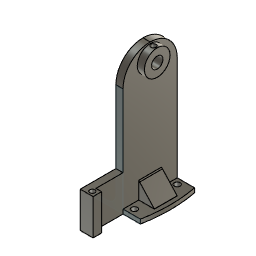
Left handle (Autodesk Fusion 360 design; units mm, degrees)
Autodesk Fusion 360 part; units mm, degrees
note: some values were not read from the file. Set by a fixed rule: which face or edge a step refers to.
sketch "Szkic1" plane through (0, 0, 0) normal (0, 0, 1) x (1, 0, 0)
  circle A0 centre (0, 0) radius 100
  line L0 (66, 19) -> (66, -19)
  line L1 (66, -19) -> (98.1784, -19)
  line L2 (66, 19) -> (98.1784, 19)
  dimension "d1" = 200
  constraint coincident A0.centre origin
  constraint coincident A0 L1.end
  constraint perpendicular L0 L1
  constraint coincident A0 L2.end
  constraint perpendicular L0 L2
  measures "d1" diameter of A0
extrude "Wyciągnięcie proste1" add sketch "Szkic1" along normal blind 3 contours A0 L0 L1 L2 picked at (77.3333, 0)
move_face "Przesuń powierzchnię1" by (-33, 0, 0) 1 faces at (77.3333, 0, 3)
move_body "Przesuń1" bodies 1 to x (1, 0, 0) y (0, 1, 0) z (0, 0, 1) at (-66, 0, 0)
sketch "Szkic2" plane through (0, 0, 3) normal (0, 0, 1) x (-1, 0, 0)
  line L0 (0, 19) -> (-32.1784, 19)
  arc A0 (-32.1784, 19) -> (-32.1784, -19) centre (66, 0) ccw
  line L1 (-32.1784, -19) -> (0, -19)
  line L2 (0, -19) -> (0, 19)
  circle A1 centre (-4, -15) radius 2.1
  circle A2 centre (-24, -15) radius 2.1
  circle A3 centre (-4, 15) radius 2.1
  circle A4 centre (-24, 15) radius 2.1
  dimension "d5" = 4.2
  dimension "d6" = 4.2
  dimension "d7" = 4.2
  dimension "d8" = 4.2
  measures "d5" diameter of A1
  measures "d6" diameter of A2
  measures "d7" diameter of A3
  measures "d8" diameter of A4
extrude "Wyciągnięcie proste2" cut sketch "Szkic2" against normal blind 3 contours A1 | A2 | A3 | A4
sketch "Szkic3" plane through (0, 0, 3) normal (0, 0, 1) x (-1, 0, 0)
  circle A0 centre (-4, 15) radius 2.1
  circle A1 centre (-24, 15) radius 2.1
  circle A2 centre (-4, -15) radius 2.1
  circle A3 centre (-24, -15) radius 2.1
  line L0 (0, 19) -> (-32.1784, 19)
  arc A4 (-32.1784, 19) -> (-32.1784, -19) centre (66, 0) ccw
  line L1 (-32.1784, -19) -> (0, -19)
  line L2 (0, -19) -> (0, 19)
  line L3 (-15, -19) -> (-20, -19)
  line L4 (-20, -19) -> (-20, 19)
  line L5 (-20, 19) -> (-15, 19)
  line L6 (-15, 19) -> (-15, -19)
  constraint horizontal L3
  constraint vertical L4
  constraint horizontal L5
  constraint vertical L6
  constraint coincident L0 L4.end
  constraint coincident L1 L3.start
extrude "Wyciągnięcie proste3" add sketch "Szkic3" along normal blind 72 contours L0 L1 L3 L4 L5 L6
extrude "Wyciągnięcie proste4" add 1 faces at (18.3333, -6.3333, 75) along direction (0, 0, 1) blind 30
extrude "Wyciągnięcie proste5" cut 1 faces at (18.3333, -6.3333, 105) along direction (0, 0, -1) blind 10
sketch "Szkic4" plane through (15, 0, 0) normal (-1, 0, 0) x (0, -1, 0)
  line L0 (19, 95) -> (-19, 95)
  line L1 (-19, 95) -> (-19, 3)
  line L2 (-19, 3) -> (19, 3)
  line L3 (19, 3) -> (19, 95)
  circle A0 centre (0, 85) radius 4
extrude "Wyciągnięcie proste6" cut sketch "Szkic4" against normal blind 5 contours A0
fillet "Zaokrąglenie1" radius 19 2 edges at (17.5, -19, 95) (17.5, 19, 95)
sketch "Szkic5" plane through (20, 0, 0) normal (1, 0, 0) x (0, 1, 0)
  circle A0 centre (0, 85) radius 4
  arc A1 (19, 76) -> (0, 95) centre (0, 76) ccw
  arc A2 (0, 95) -> (-19, 76) centre (0, 76) ccw
  line L0 (-19, 76) -> (-19, 3)
  line L1 (-19, 3) -> (19, 3)
  line L2 (19, 3) -> (19, 76)
  circle A3 centre (0, 85) radius 9
  dimension "d21" = 18
  constraint concentric A0 A3
  measures "d21" diameter of A3
extrude "Wyciągnięcie proste7" add sketch "Szkic5" along normal blind 5 contours A3
sketch "Szkic6" plane through (0, 0, 3) normal (0, 0, 1) x (-1, 0, 0)
  line L0 (-20, -19) -> (-20, 19)
  line L1 (-20, 19) -> (-32.1784, 19)
  arc A0 (-32.1784, 19) -> (-32.1784, -19) centre (66, 0) ccw
  line L2 (-32.1784, -19) -> (-20, -19)
  circle A1 centre (-24, -15) radius 2.1
  circle A2 centre (-24, 15) radius 2.1
  circle A3 through (-20.7, 0, 92.5) (-23.4, 1.5588, 92.5) (-23.4, -1.5588, 92.5)
  dimension "d24" = 3.6
extrude "Wyciągnięcie proste8" cut sketch "Szkic6" against normal blind 8 contours A3 in plane through (0, 0, 95.5) normal (0, 0, 1)
sketch "Szkic7" plane through (0, 0, 0) normal (0, 1, 0) x (1, 0, 0)
  line L0 (20, -35) -> (28, -35)
  line L1 (28, -35) -> (28, -3)
  line L2 (28, -3) -> (20, -3)
  line L3 (20, -3) -> (20, -35)
  line L4 (15, -35) -> (7, -35)
  line L5 (7, -35) -> (7, -3)
  line L6 (7, -3) -> (15, -3)
  line L7 (15, -3) -> (15, -35)
  constraint horizontal L0
  constraint vertical L1
  constraint horizontal L2
  constraint vertical L3
  constraint horizontal L4
  constraint vertical L5
  constraint horizontal L6
  constraint vertical L7
extrude "Wyciągnięcie proste9" add sketch "Szkic7" along normal mid plane 16
extrude "Wyciągnięcie proste10" cut 2 faces at (25.3333, 2.6667, 35) (9.6667, 2.6667, 35) along direction (0, 0, -1) blind 28
sketch "Szkic8" plane through (20, 0, 0) normal (1, 0, 0) x (0, 1, 0)
  line L0 (8, 7) -> (8, 3)
  line L1 (8, 3) -> (19, 3)
  line L2 (19, 3) -> (19, 76)
  arc A0 (19, 76) -> (0, 95) centre (0, 76) ccw
  arc A1 (0, 95) -> (-19, 76) centre (0, 76) ccw
  line L3 (-19, 76) -> (-19, 3)
  line L4 (-19, 3) -> (-8, 3)
  line L5 (-8, 3) -> (-8, 7)
  line L6 (-8, 7) -> (8, 7)
  circle A2 centre (0, 85) radius 9
  line L7 (-8, 7) -> (8, 7)
  line L8 (8, 7) -> (8, 35)
  line L9 (8, 35) -> (-8, 35)
  line L10 (-8, 35) -> (-8, 7)
  constraint horizontal L7
  constraint vertical L8
  constraint horizontal L9
  constraint vertical L10
  constraint coincident L5.end L6.start
extrude "Wyciągnięcie proste11" add sketch "Szkic8" along normal blind 4 and the other way blind 9 contours L6 L7 L8 L9 L10
extrude "Wyciągnięcie proste12" cut 1 faces at (11, 2.6667, 25.6667) along direction (1, 0, 0) blind 1
extrude "Wyciągnięcie proste13" cut 2 faces at (11.3333, -2.6667, 7) (9.6667, -2.6667, 7) along direction (0, 0, -1) blind 2
extrude "Wyciągnięcie proste14" add 2 faces at (14, -8, 5) (13, -8, 25.6667) along direction (0, -1, 0) blind 11
extrude "Wyciągnięcie proste15" add 2 faces at (14, 8, 5) (13, 8, 25.6667) along direction (0, 1, 0) blind 11
extrude "Wyciągnięcie proste16" cut 1 faces at (10.3333, -6.3333, 5) along direction (0, 0, -1) blind 2
extrude "Wyciągnięcie proste17" cut 1 faces at (12, -6.3333, 15) along direction (1, 0, 0) blind 3
fillet "Zaokrąglenie2" radius 6 1 edges at (15, 0, 3)
extrude "Wyciągnięcie proste18" cut 1 faces at (22.6667, 2.6667, 35) along direction (0, 0, -1) blind 20
extrude "Wyciągnięcie proste19" add 1 faces at (28, 2.6667, 5.6667) along direction (1, 0, 0) blind 3
sketch "Szkic9" plane through (0, -19, 0) normal (0, -1, 0) x (1, 0, 0)
  arc A0 (9, 3) -> (15, 9) centre (9, 9) ccw
  line L0 (9, 3) -> (0, 3)
  line L1 (0, 3) -> (0, 0)
  line L2 (0, 0) -> (32.1784, 0)
  line L3 (32.1784, 0) -> (32.1784, 3)
  line L4 (32.1784, 3) -> (20, 3)
  line L5 (20, 3) -> (20, 76)
  line L6 (20, 76) -> (15, 76)
  line L7 (15, 76) -> (15, 9)
sketch "Szkic10" plane through (15, 0, 0) normal (-1, 0, 0) x (0, -1, 0)
  circle A0 centre (0, 85) radius 4
  line L0 (-19, 9) -> (19, 9)
  line L1 (19, 9) -> (19, 76)
  arc A1 (19, 76) -> (0, 95) centre (0, 76) ccw
  arc A2 (0, 95) -> (-19, 76) centre (0, 76) ccw
  line L2 (-19, 76) -> (-19, 9)
  line L3 (0, 85) -> (0, 25)
  line L4 (0, 85) -> (19, 28.0878)
  line L5 (19, 28.0878) -> (44, 28.0878)
  line L6 (44, 28.0878) -> (44, 17.0878)
  line L7 (44, 17.0878) -> (19, 17.0878)
  line L8 (19, 17.0878) -> (19, 28.0878)
  dimension "d53" = 60
  dimension "d54" = 25
  dimension "d55" = 11
  constraint coincident A0.centre L3.start
  constraint vertical L3
  constraint coincident L1 L4.end
  constraint horizontal L5
  constraint vertical L6
  constraint horizontal L7
  constraint vertical L8
  measures "d53" distance of A0.centre L4.end
  measures "d54" distance of L4.end L5.end
  measures "d55" distance of L4.end L7.end
extrude "Wyciągnięcie proste20" add sketch "Szkic10" against normal blind 5 contours L1 L5 L6 L7 L8
sketch "Szkic11" plane through (0, 0, 28.0878) normal (0, 0, 1) x (-1, 0, 0)
  line L0 (-15, 19) -> (-15, 44)
  line L1 (-15, 44) -> (-20, 44)
  line L2 (-20, 44) -> (-20, 19)
  line L3 (-20, 19) -> (-15, 19)
  line L4 (-20, 19) -> (-20, 41)
  line L5 (-20, 41) -> (-21, 41)
  circle A0 centre (-21, 41) radius 1.8
  line L6 (-20, 44) -> (-24, 44)
  line L7 (-24, 44) -> (-24, 38)
  line L8 (-24, 38) -> (-20, 38)
  line L9 (-20, 38) -> (-20, 44)
  dimension "d58" = 3.6
  constraint coincident L2.end L3.start
  constraint coincident L2 L4.end
  constraint perpendicular L3 L4
  constraint perpendicular L2 L5
  constraint coincident L5.end A0.centre
  constraint horizontal L6
  constraint vertical L7
  constraint horizontal L8
  constraint vertical L9
  constraint coincident L1.end L2.start
  measures "d58" diameter of A0
extrude "Wyciągnięcie proste21" add sketch "Szkic11" against normal blind 11 contours L2 L4 A0 L6 L7 L8 L9 | L2 L4 A0 L9 picked at (-21.8633, 41)
extrude "Wyciągnięcie proste22" cut 1 faces at (16.6667, -33.6667, 28.0878) along direction (0, 0, -1) blind 3
sketch "Szkic12" plane through (0, 0, 25.0878) normal (0, 0, 1) x (-1, 0, 0)
  line L0 (-15, 19) -> (-15, 44)
  line L1 (-15, 44) -> (-24, 44)
  line L2 (-24, 44) -> (-24, 38)
  line L3 (-24, 38) -> (-20, 38)
  line L4 (-20, 38) -> (-20, 19)
  line L5 (-20, 19) -> (-15, 19)
  line L6 (-20.5, 19) -> (-20.5, 41)
  circle A0 centre (-20.5, 41) radius 1.8
  dimension "d63" = 3.6
  constraint perpendicular L3 L6
  constraint coincident L6.end A0.centre
  measures "d63" diameter of A0
extrude "Wyciągnięcie proste23" cut sketch "Szkic12" against normal blind 5.5 contours A0
extrude "Wyciągnięcie proste24" add 1 faces at (16.6667, -33.6667, 17.0878) along direction (0, 0, -1) blind 17.1
extrude "Wyciągnięcie proste25" add 1 faces at (16.6667, -33.6667, -0.0122) along direction (0, 0, -1) blind 2.6
extrude "Wyciągnięcie proste26" cut 1 faces at (18.3333, -19, -1.7415) along direction (0, -1, 0) blind 36.2
extrude "Wyciągnięcie proste27" cut 1 faces at (20, -40, -1.7415) along direction (1, 0, 0) blind 11
fillet "Zaokrąglenie3" radius 15 2 edges at (31, 0, 7) (24, 0, 15)
chamfer "Fazowanie1" distance 8 angle 45 1 edges at (24, 0, 7)
